Autodesk Inventor part; units mm, degrees
(part 3 of 4)
sketch "Sketch8" plane through (0, 0, 0.5) normal (0, 0, 1) x (1, 0, 0)
  circle A0 centre (6, 31.8) radius 0.9
  circle A1 centre (6, -31.8) radius 0.9
  line L0 (79.1, 6.35) -> (81.4, 6.35)
  line L1 (81.4, 6.35) -> (81.4, 7.9)
  line L2 (81.4, 7.9) -> (82.4, 7.9)
  line L3 (82.4, 7.9) -> (82.4, 5.35)
  line L4 (82.4, 5.35) -> (79.1, 5.35)
  line L5 (79.1, 5.35) -> (79.1, 6.35)
  line L6 (37.6, 36.65) -> (40.9, 36.65)
  line L7 (40.9, 36.65) -> (40.9, 35.65)
  line L8 (40.9, 35.65) -> (38.6, 35.65)
  line L9 (38.6, 35.65) -> (38.6, 34.1)
  line L10 (38.6, 34.1) -> (37.6, 34.1)
  line L11 (37.6, 34.1) -> (37.6, 36.65)
  line L12 (76.9, 36.65) -> (76.9, 35.65)
  line L13 (76.9, 35.65) -> (73.1, 35.65)
  line L14 (73.1, 35.65) -> (73.1, 36.65)
  line L15 (73.1, 36.65) -> (76.9, 36.65)
  line L16 (70.9, 6.35) -> (70.9, 5.35)
  line L17 (70.9, 5.35) -> (67.1, 5.35)
  line L18 (67.1, 5.35) -> (67.1, 6.35)
  line L19 (67.1, 6.35) -> (70.9, 6.35)
  line L20 (37.6, 16.1) -> (37.6, 19.9)
  line L21 (37.6, 19.9) -> (38.6, 19.9)
  line L22 (38.6, 19.9) -> (38.6, 16.1)
  line L23 (38.6, 16.1) -> (37.6, 16.1)
  line L24 (52.9, 36.65) -> (52.9, 35.65)
  line L25 (52.9, 35.65) -> (49.1, 35.65)
  line L26 (49.1, 35.65) -> (49.1, 36.65)
  line L27 (49.1, 36.65) -> (52.9, 36.65)
  line L28 (64.9, 36.65) -> (64.9, 35.65)
  line L29 (64.9, 35.65) -> (61.1, 35.65)
  line L30 (61.1, 35.65) -> (61.1, 36.65)
  line L31 (61.1, 36.65) -> (64.9, 36.65)
  line L32 (55.1, 6.35) -> (58.9, 6.35)
  line L33 (58.9, 6.35) -> (58.9, 5.35)
  line L34 (58.9, 5.35) -> (55.1, 5.35)
  line L35 (55.1, 5.35) -> (55.1, 6.35)
  line L36 (43.1, 6.35) -> (46.9, 6.35)
  line L37 (46.9, 6.35) -> (46.9, 5.35)
  line L38 (46.9, 5.35) -> (43.1, 5.35)
  line L39 (43.1, 5.35) -> (43.1, 6.35)
  line L40 (81.4, 25.9) -> (82.4, 25.9)
  line L41 (82.4, 25.9) -> (82.4, 22.1)
  line L42 (82.4, 22.1) -> (81.4, 22.1)
  line L43 (81.4, 22.1) -> (81.4, 25.9)
  line L44 (37.6, 28.1) -> (37.6, 31.9)
  line L45 (37.6, 31.9) -> (38.6, 31.9)
  line L46 (38.6, 31.9) -> (38.6, 28.1)
  line L47 (38.6, 28.1) -> (37.6, 28.1)
  line L48 (37.6, 10.1) -> (37.6, 13.9)
  line L49 (37.6, 13.9) -> (38.6, 13.9)
  line L50 (38.6, 13.9) -> (38.6, 10.1)
  line L51 (38.6, 10.1) -> (37.6, 10.1)
  line L52 (86.1, 14.6) -> (86.1, 13.25)
  line L53 (86.1, 13.25) -> (83.9, 13.25)
  line L54 (83.9, 13.25) -> (83.9, 14.6)
  line L55 (83.9, 14.6) -> (83.4, 14.6)
  line L56 (83.4, 14.6) -> (83.4, 15.4)
  line L57 (83.4, 15.4) -> (83.9, 15.4)
  line L58 (83.9, 15.4) -> (83.9, 16.75)
  line L59 (83.9, 16.75) -> (86.1, 16.75)
  line L60 (86.1, 16.75) -> (86.1, 15.4)
  line L61 (86.1, 15.4) -> (86.6, 15.4)
  line L62 (86.6, 15.4) -> (86.6, 14.6)
  line L63 (86.6, 14.6) -> (86.1, 14.6)
  line L64 (37.6, 22.1) -> (37.6, 25.9)
  line L65 (37.6, 25.9) -> (38.6, 25.9)
  line L66 (38.6, 25.9) -> (38.6, 22.1)
  line L67 (38.6, 22.1) -> (37.6, 22.1)
  line L68 (81.4, 31.9) -> (82.4, 31.9)
  line L69 (82.4, 31.9) -> (82.4, 28.1)
  line L70 (82.4, 28.1) -> (81.4, 28.1)
  line L71 (81.4, 28.1) -> (81.4, 31.9)
  line L72 (81.4, 13.9) -> (82.4, 13.9)
  line L73 (82.4, 13.9) -> (82.4, 10.1)
  line L74 (82.4, 10.1) -> (81.4, 10.1)
  line L75 (81.4, 10.1) -> (81.4, 13.9)
  line L76 (49.1, 6.35) -> (52.9, 6.35)
  line L77 (52.9, 6.35) -> (52.9, 5.35)
  line L78 (52.9, 5.35) -> (49.1, 5.35)
  line L79 (49.1, 5.35) -> (49.1, 6.35)
  line L80 (61.1, 6.35) -> (64.9, 6.35)
  line L81 (64.9, 6.35) -> (64.9, 5.35)
  line L82 (64.9, 5.35) -> (61.1, 5.35)
  line L83 (61.1, 5.35) -> (61.1, 6.35)
  line L84 (58.9, 36.65) -> (58.9, 35.65)
  line L85 (58.9, 35.65) -> (55.1, 35.65)
  line L86 (55.1, 35.65) -> (55.1, 36.65)
  line L87 (55.1, 36.65) -> (58.9, 36.65)
  line L88 (46.9, 36.65) -> (46.9, 35.65)
  line L89 (46.9, 35.65) -> (43.1, 35.65)
  line L90 (43.1, 35.65) -> (43.1, 36.65)
  line L91 (43.1, 36.65) -> (46.9, 36.65)
  line L92 (81.4, 19.9) -> (82.4, 19.9)
  line L93 (82.4, 19.9) -> (82.4, 16.1)
  line L94 (82.4, 16.1) -> (81.4, 16.1)
  line L95 (81.4, 16.1) -> (81.4, 19.9)
  line L96 (73.1, 6.35) -> (76.9, 6.35)
  line L97 (76.9, 6.35) -> (76.9, 5.35)
  line L98 (76.9, 5.35) -> (73.1, 5.35)
  line L99 (73.1, 5.35) -> (73.1, 6.35)
  line L100 (70.9, 36.65) -> (70.9, 35.65)
  line L101 (70.9, 35.65) -> (67.1, 35.65)
  line L102 (67.1, 35.65) -> (67.1, 36.65)
  line L103 (67.1, 36.65) -> (70.9, 36.65)
  line L104 (37.6, 5.35) -> (37.6, 7.9)
  line L105 (37.6, 7.9) -> (38.6, 7.9)
  line L106 (38.6, 7.9) -> (38.6, 6.35)
  line L107 (38.6, 6.35) -> (40.9, 6.35)
  line L108 (40.9, 6.35) -> (40.9, 5.35)
  line L109 (40.9, 5.35) -> (37.6, 5.35)
  line L110 (79.1, 35.65) -> (79.1, 36.65)
  line L111 (79.1, 36.65) -> (82.4, 36.65)
  line L112 (82.4, 36.65) -> (82.4, 34.1)
  line L113 (82.4, 34.1) -> (81.4, 34.1)
  line L114 (81.4, 34.1) -> (81.4, 35.65)
  line L115 (81.4, 35.65) -> (79.1, 35.65)
  line L116 (79.1, -33.65) -> (81.4, -33.65)
  line L117 (81.4, -33.65) -> (81.4, -32.1)
  line L118 (81.4, -32.1) -> (82.4, -32.1)
  line L119 (82.4, -32.1) -> (82.4, -34.65)
  line L120 (82.4, -34.65) -> (79.1, -34.65)
  line L121 (79.1, -34.65) -> (79.1, -33.65)
  line L122 (37.6, -3.35) -> (40.9, -3.35)
  line L123 (40.9, -3.35) -> (40.9, -4.35)
  line L124 (40.9, -4.35) -> (38.6, -4.35)
  line L125 (38.6, -4.35) -> (38.6, -5.9)
  line L126 (38.6, -5.9) -> (37.6, -5.9)
  line L127 (37.6, -5.9) -> (37.6, -3.35)
  line L128 (76.9, -3.35) -> (76.9, -4.35)
  line L129 (76.9, -4.35) -> (73.1, -4.35)
  line L130 (73.1, -4.35) -> (73.1, -3.35)
  line L131 (73.1, -3.35) -> (76.9, -3.35)
  line L132 (70.9, -33.65) -> (70.9, -34.65)
  line L133 (70.9, -34.65) -> (67.1, -34.65)
  line L134 (67.1, -34.65) -> (67.1, -33.65)
  line L135 (67.1, -33.65) -> (70.9, -33.65)
  line L136 (37.6, -23.9) -> (37.6, -20.1)
  line L137 (37.6, -20.1) -> (38.6, -20.1)
  line L138 (38.6, -20.1) -> (38.6, -23.9)
  line L139 (38.6, -23.9) -> (37.6, -23.9)
  line L140 (52.9, -3.35) -> (52.9, -4.35)
  line L141 (52.9, -4.35) -> (49.1, -4.35)
  line L142 (49.1, -4.35) -> (49.1, -3.35)
  line L143 (49.1, -3.35) -> (52.9, -3.35)
  line L144 (64.9, -3.35) -> (64.9, -4.35)
  line L145 (64.9, -4.35) -> (61.1, -4.35)
  line L146 (61.1, -4.35) -> (61.1, -3.35)
  line L147 (61.1, -3.35) -> (64.9, -3.35)
  line L148 (55.1, -33.65) -> (58.9, -33.65)
  line L149 (58.9, -33.65) -> (58.9, -34.65)
  line L150 (58.9, -34.65) -> (55.1, -34.65)
  line L151 (55.1, -34.65) -> (55.1, -33.65)
  line L152 (43.1, -33.65) -> (46.9, -33.65)
  line L153 (46.9, -33.65) -> (46.9, -34.65)
  line L154 (46.9, -34.65) -> (43.1, -34.65)
  line L155 (43.1, -34.65) -> (43.1, -33.65)
  line L156 (81.4, -14.1) -> (82.4, -14.1)
  line L157 (82.4, -14.1) -> (82.4, -17.9)
  line L158 (82.4, -17.9) -> (81.4, -17.9)
  line L159 (81.4, -17.9) -> (81.4, -14.1)
  line L160 (37.6, -11.9) -> (37.6, -8.1)
  line L161 (37.6, -8.1) -> (38.6, -8.1)
  line L162 (38.6, -8.1) -> (38.6, -11.9)
  line L163 (38.6, -11.9) -> (37.6, -11.9)
  line L164 (37.6, -29.9) -> (37.6, -26.1)
  line L165 (37.6, -26.1) -> (38.6, -26.1)
  line L166 (38.6, -26.1) -> (38.6, -29.9)
  line L167 (38.6, -29.9) -> (37.6, -29.9)
  line L168 (86.1, -25.4) -> (86.1, -26.75)
  line L169 (86.1, -26.75) -> (83.9, -26.75)
  line L170 (83.9, -26.75) -> (83.9, -25.4)
  line L171 (83.9, -25.4) -> (83.4, -25.4)
  line L172 (83.4, -25.4) -> (83.4, -24.6)
  line L173 (83.4, -24.6) -> (83.9, -24.6)
  line L174 (83.9, -24.6) -> (83.9, -23.25)
  line L175 (83.9, -23.25) -> (86.1, -23.25)
  line L176 (86.1, -23.25) -> (86.1, -24.6)
  line L177 (86.1, -24.6) -> (86.6, -24.6)
  line L178 (86.6, -24.6) -> (86.6, -25.4)
  line L179 (86.6, -25.4) -> (86.1, -25.4)
  line L180 (37.6, -17.9) -> (37.6, -14.1)
  line L181 (37.6, -14.1) -> (38.6, -14.1)
  line L182 (38.6, -14.1) -> (38.6, -17.9)
  line L183 (38.6, -17.9) -> (37.6, -17.9)
  line L184 (81.4, -8.1) -> (82.4, -8.1)
  line L185 (82.4, -8.1) -> (82.4, -11.9)
  line L186 (82.4, -11.9) -> (81.4, -11.9)
  line L187 (81.4, -11.9) -> (81.4, -8.1)
  line L188 (81.4, -26.1) -> (82.4, -26.1)
  line L189 (82.4, -26.1) -> (82.4, -29.9)
  line L190 (82.4, -29.9) -> (81.4, -29.9)
  line L191 (81.4, -29.9) -> (81.4, -26.1)
  line L192 (49.1, -33.65) -> (52.9, -33.65)
  line L193 (52.9, -33.65) -> (52.9, -34.65)
  line L194 (52.9, -34.65) -> (49.1, -34.65)
  line L195 (49.1, -34.65) -> (49.1, -33.65)
  line L196 (61.1, -33.65) -> (64.9, -33.65)
  line L197 (64.9, -33.65) -> (64.9, -34.65)
  line L198 (64.9, -34.65) -> (61.1, -34.65)
  line L199 (61.1, -34.65) -> (61.1, -33.65)
  line L200 (58.9, -3.35) -> (58.9, -4.35)
  line L201 (58.9, -4.35) -> (55.1, -4.35)
  line L202 (55.1, -4.35) -> (55.1, -3.35)
  line L203 (55.1, -3.35) -> (58.9, -3.35)
  line L204 (46.9, -3.35) -> (46.9, -4.35)
  line L205 (46.9, -4.35) -> (43.1, -4.35)
  line L206 (43.1, -4.35) -> (43.1, -3.35)
  line L207 (43.1, -3.35) -> (46.9, -3.35)
  line L208 (81.4, -20.1) -> (82.4, -20.1)
  line L209 (82.4, -20.1) -> (82.4, -23.9)
  line L210 (82.4, -23.9) -> (81.4, -23.9)
  line L211 (81.4, -23.9) -> (81.4, -20.1)
  line L212 (73.1, -33.65) -> (76.9, -33.65)
  line L213 (76.9, -33.65) -> (76.9, -34.65)
  line L214 (76.9, -34.65) -> (73.1, -34.65)
  line L215 (73.1, -34.65) -> (73.1, -33.65)
  line L216 (70.9, -3.35) -> (70.9, -4.35)
  line L217 (70.9, -4.35) -> (67.1, -4.35)
  line L218 (67.1, -4.35) -> (67.1, -3.35)
  line L219 (67.1, -3.35) -> (70.9, -3.35)
  line L220 (37.6, -34.65) -> (37.6, -32.1)
  line L221 (37.6, -32.1) -> (38.6, -32.1)
  line L222 (38.6, -32.1) -> (38.6, -33.65)
  line L223 (38.6, -33.65) -> (40.9, -33.65)
  line L224 (40.9, -33.65) -> (40.9, -34.65)
  line L225 (40.9, -34.65) -> (37.6, -34.65)
  line L226 (79.1, -4.35) -> (79.1, -3.35)
  line L227 (79.1, -3.35) -> (82.4, -3.35)
  line L228 (82.4, -3.35) -> (82.4, -5.9)
  line L229 (82.4, -5.9) -> (81.4, -5.9)
  line L230 (81.4, -5.9) -> (81.4, -4.35)
  line L231 (81.4, -4.35) -> (79.1, -4.35)
  line L232 (31.7, -27.5) -> (30.7, -27.5)
  line L233 (30.7, -27.5) -> (30.7, -25)
  line L234 (30.7, -25) -> (31.7, -25)
  line L235 (31.7, -25) -> (31.7, -27.5)
  line L236 (26.62, -27.5) -> (25.62, -27.5)
  line L237 (25.62, -27.5) -> (25.62, -25)
  line L238 (25.62, -25) -> (26.62, -25)
  line L239 (26.62, -25) -> (26.62, -27.5)
  line L240 (21.54, -27.5) -> (20.54, -27.5)
  line L241 (20.54, -27.5) -> (20.54, -25)
  line L242 (20.54, -25) -> (21.54, -25)
  line L243 (21.54, -25) -> (21.54, -27.5)
  line L244 (14.5, 8.6) -> (14.5, 9.75)
  line L245 (14.5, 9.75) -> (15.9, 9.75)
  line L246 (15.9, 9.75) -> (15.9, 8.6)
  line L247 (15.9, 8.6) -> (14.5, 8.6)
  line L248 (17.5, 7) -> (17.5, 8.15)
  line L249 (17.5, 8.15) -> (18.9, 8.15)
  line L250 (18.9, 8.15) -> (18.9, 7)
  line L251 (18.9, 7) -> (17.5, 7)
  line L252 (23.4831, 10.3536) -> (22.3831, 10.3536)
  line L253 (22.3831, 10.3536) -> (22.3831, 11.4536)
  line L254 (22.3831, 11.4536) -> (23.4831, 11.4536)
  line L255 (23.4831, 11.4536) -> (23.4831, 10.3536)
  line L256 (18.75, 11.78) -> (17.65, 11.78)
  line L257 (17.65, 11.78) -> (17.65, 12.88)
  line L258 (17.65, 12.88) -> (18.75, 12.88)
  line L259 (18.75, 12.88) -> (18.75, 11.78)
  line L260 (15.75, 11.78) -> (14.65, 11.78)
  line L261 (14.65, 11.78) -> (14.65, 12.88)
  line L262 (14.65, 12.88) -> (15.75, 12.88)
  line L263 (15.75, 12.88) -> (15.75, 11.78)
  line L264 (23.9, 6.8) -> (23.9, 7.9)
  line L265 (23.9, 7.9) -> (25, 7.9)
  line L266 (25, 7.9) -> (25, 6.8)
  line L267 (25, 6.8) -> (23.9, 6.8)
  line L268 (26.8, -3.9) -> (27.9, -3.9)
  line L269 (27.9, -3.9) -> (27.9, -5)
  line L270 (27.9, -5) -> (26.8, -5)
  line L271 (26.8, -5) -> (26.8, -3.9)
  line L272 (16.1, -6.8) -> (16.1, -7.9)
  line L273 (16.1, -7.9) -> (15, -7.9)
  line L274 (15, -7.9) -> (15, -6.8)
  line L275 (15, -6.8) -> (16.1, -6.8)
  line L276 (13.2, 5) -> (13.2, 3.9)
  line L277 (13.2, 3.9) -> (12.1, 3.9)
  line L278 (12.1, 3.9) -> (12.1, 5)
  line L279 (12.1, 5) -> (13.2, 5)
  line L280 (26.35, -3.6) -> (26.35, -3.9)
  line L281 (26.35, -3.9) -> (25.15, -3.9)
  line L282 (25.15, -3.9) -> (25.15, -3.6)
  line L283 (25.15, -3.6) -> (26.35, -3.6)
  line L284 (26.35, -3.1) -> (26.35, -3.4)
  line L285 (26.35, -3.4) -> (25.15, -3.4)
  line L286 (25.15, -3.4) -> (25.15, -3.1)
  line L287 (25.15, -3.1) -> (26.35, -3.1)
  line L288 (26.35, -2.6) -> (26.35, -2.9)
  line L289 (26.35, -2.9) -> (25.15, -2.9)
  line L290 (25.15, -2.9) -> (25.15, -2.6)
  line L291 (25.15, -2.6) -> (26.35, -2.6)
  line L292 (26.35, -2.1) -> (26.35, -2.4)
  line L293 (26.35, -2.4) -> (25.15, -2.4)
  line L294 (25.15, -2.4) -> (25.15, -2.1)
  line L295 (25.15, -2.1) -> (26.35, -2.1)
  line L296 (26.35, -1.6) -> (26.35, -1.9)
  line L297 (26.35, -1.9) -> (25.15, -1.9)
  line L298 (25.15, -1.9) -> (25.15, -1.6)
  line L299 (25.15, -1.6) -> (26.35, -1.6)
  line L300 (26.35, -1.1) -> (26.35, -1.4)
  line L301 (26.35, -1.4) -> (25.15, -1.4)
  line L302 (25.15, -1.4) -> (25.15, -1.1)
  line L303 (25.15, -1.1) -> (26.35, -1.1)
  line L304 (26.35, -0.6) -> (26.35, -0.9)
  line L305 (26.35, -0.9) -> (25.15, -0.9)
  line L306 (25.15, -0.9) -> (25.15, -0.6)
  line L307 (25.15, -0.6) -> (26.35, -0.6)
  line L308 (26.35, -0.1) -> (26.35, -0.4)
  line L309 (26.35, -0.4) -> (25.15, -0.4)
  line L310 (25.15, -0.4) -> (25.15, -0.1)
  line L311 (25.15, -0.1) -> (26.35, -0.1)
  line L312 (26.35, 0.4) -> (26.35, 0.1)
  line L313 (26.35, 0.1) -> (25.15, 0.1)
  line L314 (25.15, 0.1) -> (25.15, 0.4)
  line L315 (25.15, 0.4) -> (26.35, 0.4)
  line L316 (26.35, 0.9) -> (26.35, 0.6)
  line L317 (26.35, 0.6) -> (25.15, 0.6)
  line L318 (25.15, 0.6) -> (25.15, 0.9)
  line L319 (25.15, 0.9) -> (26.35, 0.9)
  line L320 (26.35, 1.4) -> (26.35, 1.1)
  line L321 (26.35, 1.1) -> (25.15, 1.1)
  line L322 (25.15, 1.1) -> (25.15, 1.4)
  line L323 (25.15, 1.4) -> (26.35, 1.4)
  line L324 (26.35, 1.9) -> (26.35, 1.6)
  line L325 (26.35, 1.6) -> (25.15, 1.6)
  line L326 (25.15, 1.6) -> (25.15, 1.9)
  line L327 (25.15, 1.9) -> (26.35, 1.9)
  line L328 (26.35, 2.4) -> (26.35, 2.1)
  line L329 (26.35, 2.1) -> (25.15, 2.1)
  line L330 (25.15, 2.1) -> (25.15, 2.4)
  line L331 (25.15, 2.4) -> (26.35, 2.4)
  line L332 (26.35, 2.9) -> (26.35, 2.6)
  line L333 (26.35, 2.6) -> (25.15, 2.6)
  line L334 (25.15, 2.6) -> (25.15, 2.9)
  line L335 (25.15, 2.9) -> (26.35, 2.9)
  line L336 (26.35, 3.4) -> (26.35, 3.1)
  line L337 (26.35, 3.1) -> (25.15, 3.1)
  line L338 (25.15, 3.1) -> (25.15, 3.4)
  line L339 (25.15, 3.4) -> (26.35, 3.4)
  line L340 (14.85, 3.9) -> (14.85, 3.6)
  line L341 (14.85, 3.6) -> (13.65, 3.6)
  line L342 (13.65, 3.6) -> (13.65, 3.9)
  line L343 (13.65, 3.9) -> (14.85, 3.9)
  line L344 (23.9, -5.15) -> (23.9, -6.35)
  line L345 (23.9, -6.35) -> (23.6, -6.35)
  line L346 (23.6, -6.35) -> (23.6, -5.15)
  line L347 (23.6, -5.15) -> (23.9, -5.15)
  line L348 (23.4, -5.15) -> (23.4, -6.35)
  line L349 (23.4, -6.35) -> (23.1, -6.35)
  line L350 (23.1, -6.35) -> (23.1, -5.15)
  line L351 (23.1, -5.15) -> (23.4, -5.15)
  line L352 (22.9, -5.15) -> (22.9, -6.35)
  line L353 (22.9, -6.35) -> (22.6, -6.35)
  line L354 (22.6, -6.35) -> (22.6, -5.15)
  line L355 (22.6, -5.15) -> (22.9, -5.15)
  line L356 (22.4, -5.15) -> (22.4, -6.35)
  line L357 (22.4, -6.35) -> (22.1, -6.35)
  line L358 (22.1, -6.35) -> (22.1, -5.15)
  line L359 (22.1, -5.15) -> (22.4, -5.15)
  line L360 (21.9, -5.15) -> (21.9, -6.35)
  line L361 (21.9, -6.35) -> (21.6, -6.35)
  line L362 (21.6, -6.35) -> (21.6, -5.15)
  line L363 (21.6, -5.15) -> (21.9, -5.15)
  line L364 (21.4, -5.15) -> (21.4, -6.35)
  line L365 (21.4, -6.35) -> (21.1, -6.35)
  line L366 (21.1, -6.35) -> (21.1, -5.15)
  line L367 (21.1, -5.15) -> (21.4, -5.15)
  line L368 (20.9, -5.15) -> (20.9, -6.35)
  line L369 (20.9, -6.35) -> (20.6, -6.35)
  line L370 (20.6, -6.35) -> (20.6, -5.15)
  line L371 (20.6, -5.15) -> (20.9, -5.15)
  line L372 (20.4, -5.15) -> (20.4, -6.35)
  line L373 (20.4, -6.35) -> (20.1, -6.35)
  line L374 (20.1, -6.35) -> (20.1, -5.15)
  line L375 (20.1, -5.15) -> (20.4, -5.15)
  line L376 (19.9, -5.15) -> (19.9, -6.35)
  line L377 (19.9, -6.35) -> (19.6, -6.35)
  line L378 (19.6, -6.35) -> (19.6, -5.15)
  line L379 (19.6, -5.15) -> (19.9, -5.15)
  line L380 (19.4, -5.15) -> (19.4, -6.35)
  line L381 (19.4, -6.35) -> (19.1, -6.35)
  line L382 (19.1, -6.35) -> (19.1, -5.15)
  line L383 (19.1, -5.15) -> (19.4, -5.15)
  line L384 (18.9, -5.15) -> (18.9, -6.35)
  line L385 (18.9, -6.35) -> (18.6, -6.35)
  line L386 (18.6, -6.35) -> (18.6, -5.15)
  line L387 (18.6, -5.15) -> (18.9, -5.15)
  line L388 (18.4, -5.15) -> (18.4, -6.35)
  line L389 (18.4, -6.35) -> (18.1, -6.35)
  line L390 (18.1, -6.35) -> (18.1, -5.15)
  line L391 (18.1, -5.15) -> (18.4, -5.15)
  line L392 (17.9, -5.15) -> (17.9, -6.35)
  line L393 (17.9, -6.35) -> (17.6, -6.35)
  line L394 (17.6, -6.35) -> (17.6, -5.15)
  line L395 (17.6, -5.15) -> (17.9, -5.15)
  line L396 (17.4, -5.15) -> (17.4, -6.35)
  line L397 (17.4, -6.35) -> (17.1, -6.35)
  line L398 (17.1, -6.35) -> (17.1, -5.15)
  line L399 (17.1, -5.15) -> (17.4, -5.15)
  line L400 (16.9, -5.15) -> (16.9, -6.35)
  line L401 (16.9, -6.35) -> (16.6, -6.35)
  line L402 (16.6, -6.35) -> (16.6, -5.15)
  line L403 (16.6, -5.15) -> (16.9, -5.15)
  line L404 (16.4, -5.15) -> (16.4, -6.35)
  line L405 (16.4, -6.35) -> (16.1, -6.35)
  line L406 (16.1, -6.35) -> (16.1, -5.15)
  line L407 (16.1, -5.15) -> (16.4, -5.15)
  line L408 (16.4, 6.35) -> (16.4, 5.15)
  line L409 (16.4, 5.15) -> (16.1, 5.15)
  line L410 (16.1, 5.15) -> (16.1, 6.35)
  line L411 (16.1, 6.35) -> (16.4, 6.35)
  line L412 (16.9, 6.35) -> (16.9, 5.15)
  line L413 (16.9, 5.15) -> (16.6, 5.15)
  line L414 (16.6, 5.15) -> (16.6, 6.35)
  line L415 (16.6, 6.35) -> (16.9, 6.35)
  line L416 (17.4, 6.35) -> (17.4, 5.15)
  line L417 (17.4, 5.15) -> (17.1, 5.15)
  line L418 (17.1, 5.15) -> (17.1, 6.35)
  line L419 (17.1, 6.35) -> (17.4, 6.35)
  line L420 (17.9, 6.35) -> (17.9, 5.15)
  line L421 (17.9, 5.15) -> (17.6, 5.15)
  line L422 (17.6, 5.15) -> (17.6, 6.35)
  line L423 (17.6, 6.35) -> (17.9, 6.35)
  line L424 (18.4, 6.35) -> (18.4, 5.15)
  line L425 (18.4, 5.15) -> (18.1, 5.15)
  line L426 (18.1, 5.15) -> (18.1, 6.35)
  line L427 (18.1, 6.35) -> (18.4, 6.35)
  line L428 (18.9, 6.35) -> (18.9, 5.15)
  line L429 (18.9, 5.15) -> (18.6, 5.15)
  line L430 (18.6, 5.15) -> (18.6, 6.35)
  line L431 (18.6, 6.35) -> (18.9, 6.35)
  line L432 (19.4, 6.35) -> (19.4, 5.15)
  line L433 (19.4, 5.15) -> (19.1, 5.15)
  line L434 (19.1, 5.15) -> (19.1, 6.35)
  line L435 (19.1, 6.35) -> (19.4, 6.35)
  line L436 (19.9, 6.35) -> (19.9, 5.15)
  line L437 (19.9, 5.15) -> (19.6, 5.15)
  line L438 (19.6, 5.15) -> (19.6, 6.35)
  line L439 (19.6, 6.35) -> (19.9, 6.35)
  line L440 (20.4, 6.35) -> (20.4, 5.15)
  line L441 (20.4, 5.15) -> (20.1, 5.15)
  line L442 (20.1, 5.15) -> (20.1, 6.35)
  line L443 (20.1, 6.35) -> (20.4, 6.35)
  line L444 (20.9, 6.35) -> (20.9, 5.15)
  line L445 (20.9, 5.15) -> (20.6, 5.15)
  line L446 (20.6, 5.15) -> (20.6, 6.35)
  line L447 (20.6, 6.35) -> (20.9, 6.35)
  line L448 (21.4, 6.35) -> (21.4, 5.15)
  line L449 (21.4, 5.15) -> (21.1, 5.15)
  line L450 (21.1, 5.15) -> (21.1, 6.35)
  line L451 (21.1, 6.35) -> (21.4, 6.35)
  line L452 (21.9, 6.35) -> (21.9, 5.15)
  line L453 (21.9, 5.15) -> (21.6, 5.15)
  line L454 (21.6, 5.15) -> (21.6, 6.35)
  line L455 (21.6, 6.35) -> (21.9, 6.35)
  line L456 (22.4, 6.35) -> (22.4, 5.15)
  line L457 (22.4, 5.15) -> (22.1, 5.15)
  line L458 (22.1, 5.15) -> (22.1, 6.35)
  line L459 (22.1, 6.35) -> (22.4, 6.35)
  line L460 (22.9, 6.35) -> (22.9, 5.15)
  line L461 (22.9, 5.15) -> (22.6, 5.15)
  line L462 (22.6, 5.15) -> (22.6, 6.35)
  line L463 (22.6, 6.35) -> (22.9, 6.35)
  line L464 (23.4, 6.35) -> (23.4, 5.15)
  line L465 (23.4, 5.15) -> (23.1, 5.15)
  line L466 (23.1, 5.15) -> (23.1, 6.35)
  line L467 (23.1, 6.35) -> (23.4, 6.35)
  line L468 (23.9, 6.35) -> (23.9, 5.15)
  line L469 (23.9, 5.15) -> (23.6, 5.15)
  line L470 (23.6, 5.15) -> (23.6, 6.35)
  line L471 (23.6, 6.35) -> (23.9, 6.35)
  line L472 (26.35, 3.9) -> (26.35, 3.6)
  line L473 (26.35, 3.6) -> (25.15, 3.6)
  line L474 (25.15, 3.6) -> (25.15, 3.9)
  line L475 (25.15, 3.9) -> (26.35, 3.9)
  line L476 (14.85, 3.1) -> (13.65, 3.1)
  line L477 (13.65, 3.1) -> (13.65, 3.4)
  line L478 (13.65, 3.4) -> (14.85, 3.4)
  line L479 (14.85, 3.4) -> (14.85, 3.1)
  line L480 (14.85, 2.6) -> (13.65, 2.6)
  line L481 (13.65, 2.6) -> (13.65, 2.9)
  line L482 (13.65, 2.9) -> (14.85, 2.9)
  line L483 (14.85, 2.9) -> (14.85, 2.6)
  line L484 (14.85, 2.1) -> (13.65, 2.1)
  line L485 (13.65, 2.1) -> (13.65, 2.4)
  line L486 (13.65, 2.4) -> (14.85, 2.4)
  line L487 (14.85, 2.4) -> (14.85, 2.1)
  line L488 (14.85, 1.6) -> (13.65, 1.6)
  line L489 (13.65, 1.6) -> (13.65, 1.9)
  line L490 (13.65, 1.9) -> (14.85, 1.9)
  line L491 (14.85, 1.9) -> (14.85, 1.6)
  line L492 (14.85, 1.1) -> (13.65, 1.1)
  line L493 (13.65, 1.1) -> (13.65, 1.4)
  line L494 (13.65, 1.4) -> (14.85, 1.4)
  line L495 (14.85, 1.4) -> (14.85, 1.1)
  line L496 (14.85, 0.6) -> (13.65, 0.6)
  line L497 (13.65, 0.6) -> (13.65, 0.9)
  line L498 (13.65, 0.9) -> (14.85, 0.9)
  line L499 (14.85, 0.9) -> (14.85, 0.6)
  line L500 (14.85, 0.1) -> (13.65, 0.1)
  line L501 (13.65, 0.1) -> (13.65, 0.4)
  line L502 (13.65, 0.4) -> (14.85, 0.4)
  line L503 (14.85, 0.4) -> (14.85, 0.1)
  line L504 (14.85, -0.4) -> (13.65, -0.4)
  line L505 (13.65, -0.4) -> (13.65, -0.1)
  line L506 (13.65, -0.1) -> (14.85, -0.1)
  line L507 (14.85, -0.1) -> (14.85, -0.4)
  line L508 (14.85, -0.9) -> (13.65, -0.9)
  line L509 (13.65, -0.9) -> (13.65, -0.6)
  line L510 (13.65, -0.6) -> (14.85, -0.6)
  line L511 (14.85, -0.6) -> (14.85, -0.9)
  line L512 (14.85, -1.4) -> (13.65, -1.4)
  line L513 (13.65, -1.4) -> (13.65, -1.1)
  line L514 (13.65, -1.1) -> (14.85, -1.1)
  line L515 (14.85, -1.1) -> (14.85, -1.4)
  line L516 (14.85, -1.9) -> (13.65, -1.9)
  line L517 (13.65, -1.9) -> (13.65, -1.6)
  line L518 (13.65, -1.6) -> (14.85, -1.6)
  line L519 (14.85, -1.6) -> (14.85, -1.9)
  line L520 (14.85, -2.4) -> (13.65, -2.4)
  line L521 (13.65, -2.4) -> (13.65, -2.1)
  line L522 (13.65, -2.1) -> (14.85, -2.1)
  line L523 (14.85, -2.1) -> (14.85, -2.4)
  line L524 (14.85, -2.9) -> (13.65, -2.9)
  line L525 (13.65, -2.9) -> (13.65, -2.6)
  line L526 (13.65, -2.6) -> (14.85, -2.6)
  line L527 (14.85, -2.6) -> (14.85, -2.9)
  line L528 (14.85, -3.4) -> (13.65, -3.4)
  line L529 (13.65, -3.4) -> (13.65, -3.1)
  line L530 (13.65, -3.1) -> (14.85, -3.1)
  line L531 (14.85, -3.1) -> (14.85, -3.4)
  line L532 (14.85, -3.9) -> (13.65, -3.9)
  line L533 (13.65, -3.9) -> (13.65, -3.6)
  line L534 (13.65, -3.6) -> (14.85, -3.6)
  line L535 (14.85, -3.6) -> (14.85, -3.9)
  line L536 (13.2, 6.73) -> (13.2, 5.63)
  line L537 (13.2, 5.63) -> (12.1, 5.63)
  line L538 (12.1, 5.63) -> (12.1, 6.73)
  line L539 (12.1, 6.73) -> (13.2, 6.73)
  line L540 (14.37, -6.8) -> (14.37, -7.9)
  line L541 (14.37, -7.9) -> (13.27, -7.9)
  line L542 (13.27, -7.9) -> (13.27, -6.8)
  line L543 (13.27, -6.8) -> (14.37, -6.8)
  line L544 (26.8, -5.63) -> (27.9, -5.63)
  line L545 (27.9, -5.63) -> (27.9, -6.73)
  line L546 (27.9, -6.73) -> (26.8, -6.73)
  line L547 (26.8, -6.73) -> (26.8, -5.63)
  line L548 (25.63, 6.8) -> (25.63, 7.9)
  line L549 (25.63, 7.9) -> (26.73, 7.9)
  line L550 (26.73, 7.9) -> (26.73, 6.8)
  line L551 (26.73, 6.8) -> (25.63, 6.8)
  line L552 (15.75, 10.05) -> (14.65, 10.05)
  line L553 (14.65, 10.05) -> (14.65, 11.15)
  line L554 (14.65, 11.15) -> (15.75, 11.15)
  line L555 (15.75, 11.15) -> (15.75, 10.05)
  line L556 (18.75, 10.05) -> (17.65, 10.05)
  line L557 (17.65, 10.05) -> (17.65, 11.15)
  line L558 (17.65, 11.15) -> (18.75, 11.15)
  line L559 (18.75, 11.15) -> (18.75, 10.05)
  line L560 (25.2131, 10.3536) -> (24.1131, 10.3536)
  line L561 (24.1131, 10.3536) -> (24.1131, 11.4536)
  line L562 (24.1131, 11.4536) -> (25.2131, 11.4536)
  line L563 (25.2131, 11.4536) -> (25.2131, 10.3536)
  line L564 (18.9, 9.75) -> (18.9, 8.6)
  line L565 (18.9, 8.6) -> (17.5, 8.6)
  line L566 (17.5, 8.6) -> (17.5, 9.75)
  line L567 (17.5, 9.75) -> (18.9, 9.75)
  line L568 (14.5, 7) -> (14.5, 8.15)
  line L569 (14.5, 8.15) -> (15.9, 8.15)
  line L570 (15.9, 8.15) -> (15.9, 7)
  line L571 (15.9, 7) -> (14.5, 7)
  line L572 (19, -25) -> (19, -27.5)
  line L573 (19, -27.5) -> (18, -27.5)
  line L574 (18, -27.5) -> (18, -25)
  line L575 (18, -25) -> (19, -25)
  line L576 (24.08, -27.5) -> (23.08, -27.5)
  line L577 (23.08, -27.5) -> (23.08, -25)
  line L578 (23.08, -25) -> (24.08, -25)
  line L579 (24.08, -25) -> (24.08, -27.5)
  line L580 (29.16, -27.5) -> (28.16, -27.5)
  line L581 (28.16, -27.5) -> (28.16, -25)
  line L582 (28.16, -25) -> (29.16, -25)
  line L583 (29.16, -25) -> (29.16, -27.5)
  line L584 (2.8, -31.125) -> (2.8, -31.575)
  line L585 (2.8, -31.575) -> (0.25, -31.575)
  line L586 (0.25, -31.575) -> (0.25, -31.125)
  line L587 (0.25, -31.125) -> (2.8, -31.125)
  line L588 (2.8, -29.925) -> (2.8, -30.375)
  line L589 (2.8, -30.375) -> (0.25, -30.375)
  line L590 (0.25, -30.375) -> (0.25, -29.925)
  line L591 (0.25, -29.925) -> (2.8, -29.925)
  line L592 (2.8, -28.725) -> (2.8, -29.175)
  line L593 (2.8, -29.175) -> (0.25, -29.175)
  line L594 (0.25, -29.175) -> (0.25, -28.725)
  line L595 (0.25, -28.725) -> (2.8, -28.725)
  line L596 (2.8, -27.525) -> (2.8, -27.975)
  line L597 (2.8, -27.975) -> (0.25, -27.975)
  line L598 (0.25, -27.975) -> (0.25, -27.525)
  line L599 (0.25, -27.525) -> (2.8, -27.525)
  line L600 (2.8, -26.325) -> (2.8, -26.775)
  line L601 (2.8, -26.775) -> (0.25, -26.775)
  line L602 (0.25, -26.775) -> (0.25, -26.325)
  line L603 (0.25, -26.325) -> (2.8, -26.325)
  line L604 (2.8, -25.125) -> (2.8, -25.575)
  line L605 (2.8, -25.575) -> (0.25, -25.575)
  line L606 (0.25, -25.575) -> (0.25, -25.125)
  line L607 (0.25, -25.125) -> (2.8, -25.125)
  line L608 (2.8, -23.925) -> (2.8, -24.375)
  line L609 (2.8, -24.375) -> (0.25, -24.375)
  line L610 (0.25, -24.375) -> (0.25, -23.925)
  line L611 (0.25, -23.925) -> (2.8, -23.925)
  line L612 (2.8, -22.725) -> (2.8, -23.175)
  line L613 (2.8, -23.175) -> (0.25, -23.175)
  line L614 (0.25, -23.175) -> (0.25, -22.725)
  line L615 (0.25, -22.725) -> (2.8, -22.725)
  line L616 (2.8, -21.525) -> (2.8, -21.975)
  line L617 (2.8, -21.975) -> (0.25, -21.975)
  line L618 (0.25, -21.975) -> (0.25, -21.525)
  line L619 (0.25, -21.525) -> (2.8, -21.525)
  line L620 (2.8, -20.325) -> (2.8, -20.775)
  line L621 (2.8, -20.775) -> (0.25, -20.775)
  line L622 (0.25, -20.775) -> (0.25, -20.325)
  line L623 (0.25, -20.325) -> (2.8, -20.325)
  line L624 (2.8, -19.125) -> (2.8, -19.575)
  line L625 (2.8, -19.575) -> (0.25, -19.575)
  line L626 (0.25, -19.575) -> (0.25, -19.125)
  line L627 (0.25, -19.125) -> (2.8, -19.125)
  line L628 (2.8, -17.925) -> (2.8, -18.375)
  line L629 (2.8, -18.375) -> (0.25, -18.375)
  line L630 (0.25, -18.375) -> (0.25, -17.925)
  line L631 (0.25, -17.925) -> (2.8, -17.925)
  line L632 (2.8, -16.725) -> (2.8, -17.175)
  line L633 (2.8, -17.175) -> (0.25, -17.175)
  line L634 (0.25, -17.175) -> (0.25, -16.725)
  line L635 (0.25, -16.725) -> (2.8, -16.725)
  line L636 (2.8, -15.525) -> (2.8, -15.975)
  line L637 (2.8, -15.975) -> (0.25, -15.975)
  line L638 (0.25, -15.975) -> (0.25, -15.525)
  line L639 (0.25, -15.525) -> (2.8, -15.525)
  line L640 (2.8, -14.325) -> (2.8, -14.775)
  line L641 (2.8, -14.775) -> (0.25, -14.775)
  line L642 (0.25, -14.775) -> (0.25, -14.325)
  line L643 (0.25, -14.325) -> (2.8, -14.325)
  line L644 (2.8, -13.125) -> (2.8, -13.575)
  line L645 (2.8, -13.575) -> (0.25, -13.575)
  line L646 (0.25, -13.575) -> (0.25, -13.125)
  line L647 (0.25, -13.125) -> (2.8, -13.125)
  line L648 (2.8, -11.925) -> (2.8, -12.375)
  line L649 (2.8, -12.375) -> (0.25, -12.375)
  line L650 (0.25, -12.375) -> (0.25, -11.925)
  line L651 (0.25, -11.925) -> (2.8, -11.925)
  line L652 (2.8, -10.725) -> (2.8, -11.175)
  line L653 (2.8, -11.175) -> (0.25, -11.175)
  line L654 (0.25, -11.175) -> (0.25, -10.725)
  line L655 (0.25, -10.725) -> (2.8, -10.725)
  line L656 (2.8, -9.525) -> (2.8, -9.975)
  line L657 (2.8, -9.975) -> (0.25, -9.975)
  line L658 (0.25, -9.975) -> (0.25, -9.525)
  line L659 (0.25, -9.525) -> (2.8, -9.525)
  line L660 (2.8, -8.325) -> (2.8, -8.775)
  line L661 (2.8, -8.775) -> (0.25, -8.775)
  line L662 (0.25, -8.775) -> (0.25, -8.325)
  line L663 (0.25, -8.325) -> (2.8, -8.325)
  line L664 (2.8, -7.125) -> (2.8, -7.575)
  line L665 (2.8, -7.575) -> (0.25, -7.575)
  line L666 (0.25, -7.575) -> (0.25, -7.125)
  line L667 (0.25, -7.125) -> (2.8, -7.125)
  line L668 (2.8, -5.925) -> (2.8, -6.375)
  line L669 (2.8, -6.375) -> (0.25, -6.375)
  line L670 (0.25, -6.375) -> (0.25, -5.925)
  line L671 (0.25, -5.925) -> (2.8, -5.925)
  line L672 (2.8, -4.725) -> (2.8, -5.175)
  line L673 (2.8, -5.175) -> (0.25, -5.175)
  line L674 (0.25, -5.175) -> (0.25, -4.725)
  line L675 (0.25, -4.725) -> (2.8, -4.725)
  line L676 (2.8, -3.525) -> (2.8, -3.975)
  line L677 (2.8, -3.975) -> (0.25, -3.975)
  line L678 (0.25, -3.975) -> (0.25, -3.525)
  line L679 (0.25, -3.525) -> (2.8, -3.525)
  line L680 (2.8, -2.325) -> (2.8, -2.775)
  line L681 (2.8, -2.775) -> (0.25, -2.775)
  line L682 (0.25, -2.775) -> (0.25, -2.325)
  line L683 (0.25, -2.325) -> (2.8, -2.325)
  line L684 (2.8, -1.125) -> (2.8, -1.575)
  line L685 (2.8, -1.575) -> (0.25, -1.575)
  line L686 (0.25, -1.575) -> (0.25, -1.125)
  line L687 (0.25, -1.125) -> (2.8, -1.125)
  line L688 (2.8, 0.075) -> (2.8, -0.375)
  line L689 (2.8, -0.375) -> (0.25, -0.375)
  line L690 (0.25, -0.375) -> (0.25, 0.075)
  line L691 (0.25, 0.075) -> (2.8, 0.075)
  line L692 (2.8, 1.275) -> (2.8, 0.825)
  line L693 (2.8, 0.825) -> (0.25, 0.825)
  line L694 (0.25, 0.825) -> (0.25, 1.275)
  line L695 (0.25, 1.275) -> (2.8, 1.275)
  line L696 (2.8, 2.475) -> (2.8, 2.025)
  line L697 (2.8, 2.025) -> (0.25, 2.025)
  line L698 (0.25, 2.025) -> (0.25, 2.475)
  line L699 (0.25, 2.475) -> (2.8, 2.475)
  line L700 (2.8, 3.675) -> (2.8, 3.225)
  line L701 (2.8, 3.225) -> (0.25, 3.225)
  line L702 (0.25, 3.225) -> (0.25, 3.675)
  line L703 (0.25, 3.675) -> (2.8, 3.675)
  line L704 (2.8, 4.875) -> (2.8, 4.425)
  line L705 (2.8, 4.425) -> (0.25, 4.425)
  line L706 (0.25, 4.425) -> (0.25, 4.875)
  line L707 (0.25, 4.875) -> (2.8, 4.875)
  line L708 (2.8, 6.075) -> (2.8, 5.625)
  line L709 (2.8, 5.625) -> (0.25, 5.625)
  line L710 (0.25, 5.625) -> (0.25, 6.075)
  line L711 (0.25, 6.075) -> (2.8, 6.075)
  line L712 (2.8, 7.275) -> (2.8, 6.825)
  line L713 (2.8, 6.825) -> (0.25, 6.825)
  line L714 (0.25, 6.825) -> (0.25, 7.275)
  line L715 (0.25, 7.275) -> (2.8, 7.275)
  line L716 (2.8, 8.475) -> (2.8, 8.025)
  line L717 (2.8, 8.025) -> (0.25, 8.025)
  line L718 (0.25, 8.025) -> (0.25, 8.475)
  line L719 (0.25, 8.475) -> (2.8, 8.475)
  line L720 (2.8, 9.675) -> (2.8, 9.225)
  line L721 (2.8, 9.225) -> (0.25, 9.225)
  line L722 (0.25, 9.225) -> (0.25, 9.675)
  line L723 (0.25, 9.675) -> (2.8, 9.675)
  line L724 (2.8, 10.875) -> (2.8, 10.425)
  line L725 (2.8, 10.425) -> (0.25, 10.425)
  line L726 (0.25, 10.425) -> (0.25, 10.875)
  line L727 (0.25, 10.875) -> (2.8, 10.875)
  line L728 (2.8, 12.075) -> (2.8, 11.625)
  line L729 (2.8, 11.625) -> (0.25, 11.625)
  line L730 (0.25, 11.625) -> (0.25, 12.075)
  line L731 (0.25, 12.075) -> (2.8, 12.075)
  line L732 (2.8, 13.275) -> (2.8, 12.825)
  line L733 (2.8, 12.825) -> (0.25, 12.825)
  line L734 (0.25, 12.825) -> (0.25, 13.275)
  line L735 (0.25, 13.275) -> (2.8, 13.275)
  line L736 (2.8, 14.475) -> (2.8, 14.025)
  line L737 (2.8, 14.025) -> (0.25, 14.025)
  line L738 (0.25, 14.025) -> (0.25, 14.475)
  line L739 (0.25, 14.475) -> (2.8, 14.475)
  line L740 (2.8, 15.675) -> (2.8, 15.225)
  line L741 (2.8, 15.225) -> (0.25, 15.225)
  line L742 (0.25, 15.225) -> (0.25, 15.675)
  line L743 (0.25, 15.675) -> (2.8, 15.675)
  line L744 (2.8, 21.075) -> (2.8, 20.625)
  line L745 (2.8, 20.625) -> (0.25, 20.625)
  line L746 (0.25, 20.625) -> (0.25, 21.075)
  line L747 (0.25, 21.075) -> (2.8, 21.075)
  line L748 (2.8, 22.275) -> (2.8, 21.825)
  line L749 (2.8, 21.825) -> (0.25, 21.825)
  line L750 (0.25, 21.825) -> (0.25, 22.275)
  line L751 (0.25, 22.275) -> (2.8, 22.275)
  line L752 (2.8, 23.475) -> (2.8, 23.025)
  line L753 (2.8, 23.025) -> (0.25, 23.025)
  line L754 (0.25, 23.025) -> (0.25, 23.475)
  line L755 (0.25, 23.475) -> (2.8, 23.475)
  line L756 (2.8, 24.675) -> (2.8, 24.225)
  line L757 (2.8, 24.225) -> (0.25, 24.225)
  line L758 (0.25, 24.225) -> (0.25, 24.675)
  line L759 (0.25, 24.675) -> (2.8, 24.675)
  line L760 (2.8, 25.875) -> (2.8, 25.425)
  line L761 (2.8, 25.425) -> (0.25, 25.425)
  line L762 (0.25, 25.425) -> (0.25, 25.875)
  line L763 (0.25, 25.875) -> (2.8, 25.875)
  line L764 (2.8, 27.075) -> (2.8, 26.625)
  line L765 (2.8, 26.625) -> (0.25, 26.625)
  line L766 (0.25, 26.625) -> (0.25, 27.075)
  line L767 (0.25, 27.075) -> (2.8, 27.075)
  line L768 (2.8, 28.275) -> (2.8, 27.825)
  line L769 (2.8, 27.825) -> (0.25, 27.825)
  line L770 (0.25, 27.825) -> (0.25, 28.275)
  line L771 (0.25, 28.275) -> (2.8, 28.275)
  line L772 (2.8, 29.475) -> (2.8, 29.025)
  line L773 (2.8, 29.025) -> (0.25, 29.025)
  line L774 (0.25, 29.025) -> (0.25, 29.475)
  line L775 (0.25, 29.475) -> (2.8, 29.475)
  line L776 (2.8, 30.675) -> (2.8, 30.225)
  line L777 (2.8, 30.225) -> (0.25, 30.225)
  line L778 (0.25, 30.225) -> (0.25, 30.675)
  line L779 (0.25, 30.675) -> (2.8, 30.675)
  line L780 (2.8, 16.275) -> (2.8, 15.825)
  line L781 (2.8, 15.825) -> (0.25, 15.825)
  line L782 (0.25, 15.825) -> (0.25, 16.275)
  line L783 (0.25, 16.275) -> (2.8, 16.275)
  line L784 (2.8, 31.875) -> (2.8, 31.425)
  line L785 (2.8, 31.425) -> (0.25, 31.425)
  line L786 (0.25, 31.425) -> (0.25, 31.875)
  line L787 (0.25, 31.875) -> (2.8, 31.875)
  line L788 (2.8, 31.275) -> (2.8, 30.825)
  line L789 (2.8, 30.825) -> (0.25, 30.825)
  line L790 (0.25, 30.825) -> (0.25, 31.275)
  line L791 (0.25, 31.275) -> (2.8, 31.275)
  line L792 (2.8, 30.075) -> (2.8, 29.625)
  line L793 (2.8, 29.625) -> (0.25, 29.625)
  line L794 (0.25, 29.625) -> (0.25, 30.075)
  line L795 (0.25, 30.075) -> (2.8, 30.075)
  line L796 (2.8, 28.875) -> (2.8, 28.425)
  line L797 (2.8, 28.425) -> (0.25, 28.425)
  line L798 (0.25, 28.425) -> (0.25, 28.875)
  line L799 (0.25, 28.875) -> (2.8, 28.875)
  line L800 (2.8, 27.675) -> (2.8, 27.225)
  line L801 (2.8, 27.225) -> (0.25, 27.225)
  line L802 (0.25, 27.225) -> (0.25, 27.675)
  line L803 (0.25, 27.675) -> (2.8, 27.675)
  line L804 (2.8, 26.475) -> (2.8, 26.025)
  line L805 (2.8, 26.025) -> (0.25, 26.025)
  line L806 (0.25, 26.025) -> (0.25, 26.475)
  line L807 (0.25, 26.475) -> (2.8, 26.475)
  line L808 (2.8, 25.275) -> (2.8, 24.825)
  line L809 (2.8, 24.825) -> (0.25, 24.825)
  line L810 (0.25, 24.825) -> (0.25, 25.275)
  line L811 (0.25, 25.275) -> (2.8, 25.275)
  line L812 (2.8, 24.075) -> (2.8, 23.625)
  line L813 (2.8, 23.625) -> (0.25, 23.625)
  line L814 (0.25, 23.625) -> (0.25, 24.075)
  line L815 (0.25, 24.075) -> (2.8, 24.075)
  line L816 (2.8, 22.875) -> (2.8, 22.425)
  line L817 (2.8, 22.425) -> (0.25, 22.425)
  line L818 (0.25, 22.425) -> (0.25, 22.875)
  line L819 (0.25, 22.875) -> (2.8, 22.875)
  line L820 (2.8, 21.675) -> (2.8, 21.225)
  line L821 (2.8, 21.225) -> (0.25, 21.225)
  line L822 (0.25, 21.225) -> (0.25, 21.675)
  line L823 (0.25, 21.675) -> (2.8, 21.675)
  line L824 (2.8, 20.475) -> (2.8, 20.025)
  line L825 (2.8, 20.025) -> (0.25, 20.025)
  line L826 (0.25, 20.025) -> (0.25, 20.475)
  line L827 (0.25, 20.475) -> (2.8, 20.475)
  line L828 (2.8, 15.075) -> (2.8, 14.625)
  line L829 (2.8, 14.625) -> (0.25, 14.625)
  line L830 (0.25, 14.625) -> (0.25, 15.075)
  line L831 (0.25, 15.075) -> (2.8, 15.075)
  line L832 (2.8, 13.875) -> (2.8, 13.425)
  line L833 (2.8, 13.425) -> (0.25, 13.425)
  line L834 (0.25, 13.425) -> (0.25, 13.875)
  line L835 (0.25, 13.875) -> (2.8, 13.875)
  line L836 (2.8, 12.675) -> (2.8, 12.225)
  line L837 (2.8, 12.225) -> (0.25, 12.225)
  line L838 (0.25, 12.225) -> (0.25, 12.675)
  line L839 (0.25, 12.675) -> (2.8, 12.675)
  line L840 (2.8, 11.475) -> (2.8, 11.025)
  line L841 (2.8, 11.025) -> (0.25, 11.025)
  line L842 (0.25, 11.025) -> (0.25, 11.475)
  line L843 (0.25, 11.475) -> (2.8, 11.475)
  line L844 (2.8, 10.275) -> (2.8, 9.825)
  line L845 (2.8, 9.825) -> (0.25, 9.825)
  line L846 (0.25, 9.825) -> (0.25, 10.275)
  line L847 (0.25, 10.275) -> (2.8, 10.275)
  line L848 (2.8, 9.075) -> (2.8, 8.625)
  line L849 (2.8, 8.625) -> (0.25, 8.625)
  line L850 (0.25, 8.625) -> (0.25, 9.075)
  line L851 (0.25, 9.075) -> (2.8, 9.075)
  line L852 (2.8, 7.875) -> (2.8, 7.425)
  line L853 (2.8, 7.425) -> (0.25, 7.425)
  line L854 (0.25, 7.425) -> (0.25, 7.875)
  line L855 (0.25, 7.875) -> (2.8, 7.875)
  line L856 (2.8, 6.675) -> (2.8, 6.225)
  line L857 (2.8, 6.225) -> (0.25, 6.225)
  line L858 (0.25, 6.225) -> (0.25, 6.675)
  line L859 (0.25, 6.675) -> (2.8, 6.675)
  line L860 (2.8, 5.475) -> (2.8, 5.025)
  line L861 (2.8, 5.025) -> (0.25, 5.025)
  line L862 (0.25, 5.025) -> (0.25, 5.475)
  line L863 (0.25, 5.475) -> (2.8, 5.475)
  line L864 (2.8, 4.275) -> (2.8, 3.825)
  line L865 (2.8, 3.825) -> (0.25, 3.825)
  line L866 (0.25, 3.825) -> (0.25, 4.275)
  line L867 (0.25, 4.275) -> (2.8, 4.275)
  line L868 (2.8, 3.075) -> (2.8, 2.625)
  line L869 (2.8, 2.625) -> (0.25, 2.625)
  line L870 (0.25, 2.625) -> (0.25, 3.075)
  line L871 (0.25, 3.075) -> (2.8, 3.075)
  line L872 (2.8, 1.875) -> (2.8, 1.425)
  line L873 (2.8, 1.425) -> (0.25, 1.425)
  line L874 (0.25, 1.425) -> (0.25, 1.875)
  line L875 (0.25, 1.875) -> (2.8, 1.875)
  line L876 (2.8, 0.675) -> (2.8, 0.225)
  line L877 (2.8, 0.225) -> (0.25, 0.225)
  line L878 (0.25, 0.225) -> (0.25, 0.675)
  line L879 (0.25, 0.675) -> (2.8, 0.675)
  line L880 (2.8, -0.525) -> (2.8, -0.975)
  line L881 (2.8, -0.975) -> (0.25, -0.975)
  line L882 (0.25, -0.975) -> (0.25, -0.525)
  line L883 (0.25, -0.525) -> (2.8, -0.525)
  line L884 (2.8, -1.725) -> (2.8, -2.175)
  line L885 (2.8, -2.175) -> (0.25, -2.175)
  line L886 (0.25, -2.175) -> (0.25, -1.725)
  line L887 (0.25, -1.725) -> (2.8, -1.725)
  line L888 (2.8, -2.925) -> (2.8, -3.375)
  line L889 (2.8, -3.375) -> (0.25, -3.375)
  line L890 (0.25, -3.375) -> (0.25, -2.925)
  line L891 (0.25, -2.925) -> (2.8, -2.925)
  line L892 (2.8, -4.125) -> (2.8, -4.575)
  line L893 (2.8, -4.575) -> (0.25, -4.575)
  line L894 (0.25, -4.575) -> (0.25, -4.125)
  line L895 (0.25, -4.125) -> (2.8, -4.125)
  line L896 (2.8, -5.325) -> (2.8, -5.775)
  line L897 (2.8, -5.775) -> (0.25, -5.775)
  line L898 (0.25, -5.775) -> (0.25, -5.325)
  line L899 (0.25, -5.325) -> (2.8, -5.325)
  line L900 (2.8, -6.525) -> (2.8, -6.975)
  line L901 (2.8, -6.975) -> (0.25, -6.975)
  line L902 (0.25, -6.975) -> (0.25, -6.525)
  line L903 (0.25, -6.525) -> (2.8, -6.525)
  line L904 (2.8, -7.725) -> (2.8, -8.175)
  line L905 (2.8, -8.175) -> (0.25, -8.175)
  line L906 (0.25, -8.175) -> (0.25, -7.725)
  line L907 (0.25, -7.725) -> (2.8, -7.725)
  line L908 (2.8, -8.925) -> (2.8, -9.375)
  line L909 (2.8, -9.375) -> (0.25, -9.375)
  line L910 (0.25, -9.375) -> (0.25, -8.925)
  line L911 (0.25, -8.925) -> (2.8, -8.925)
  line L912 (2.8, -10.125) -> (2.8, -10.575)
  line L913 (2.8, -10.575) -> (0.25, -10.575)
  line L914 (0.25, -10.575) -> (0.25, -10.125)
  line L915 (0.25, -10.125) -> (2.8, -10.125)
  line L916 (2.8, -11.325) -> (2.8, -11.775)
  line L917 (2.8, -11.775) -> (0.25, -11.775)
  line L918 (0.25, -11.775) -> (0.25, -11.325)
  line L919 (0.25, -11.325) -> (2.8, -11.325)
  line L920 (2.8, -12.525) -> (2.8, -12.975)
  line L921 (2.8, -12.975) -> (0.25, -12.975)
  line L922 (0.25, -12.975) -> (0.25, -12.525)
  line L923 (0.25, -12.525) -> (2.8, -12.525)
  line L924 (2.8, -13.725) -> (2.8, -14.175)
  line L925 (2.8, -14.175) -> (0.25, -14.175)
  line L926 (0.25, -14.175) -> (0.25, -13.725)
  line L927 (0.25, -13.725) -> (2.8, -13.725)
  line L928 (2.8, -14.925) -> (2.8, -15.375)
  line L929 (2.8, -15.375) -> (0.25, -15.375)
  line L930 (0.25, -15.375) -> (0.25, -14.925)
  line L931 (0.25, -14.925) -> (2.8, -14.925)
  line L932 (2.8, -16.125) -> (2.8, -16.575)
  line L933 (2.8, -16.575) -> (0.25, -16.575)
  line L934 (0.25, -16.575) -> (0.25, -16.125)
  line L935 (0.25, -16.125) -> (2.8, -16.125)
  line L936 (2.8, -17.325) -> (2.8, -17.775)
  line L937 (2.8, -17.775) -> (0.25, -17.775)
  line L938 (0.25, -17.775) -> (0.25, -17.325)
  line L939 (0.25, -17.325) -> (2.8, -17.325)
  line L940 (2.8, -18.525) -> (2.8, -18.975)
  line L941 (2.8, -18.975) -> (0.25, -18.975)
  line L942 (0.25, -18.975) -> (0.25, -18.525)
  line L943 (0.25, -18.525) -> (2.8, -18.525)
  line L944 (2.8, -19.725) -> (2.8, -20.175)
  line L945 (2.8, -20.175) -> (0.25, -20.175)
  line L946 (0.25, -20.175) -> (0.25, -19.725)
  line L947 (0.25, -19.725) -> (2.8, -19.725)
  line L948 (2.8, -20.925) -> (2.8, -21.375)
  line L949 (2.8, -21.375) -> (0.25, -21.375)
  line L950 (0.25, -21.375) -> (0.25, -20.925)
  line L951 (0.25, -20.925) -> (2.8, -20.925)
  line L952 (2.8, -22.125) -> (2.8, -22.575)
  line L953 (2.8, -22.575) -> (0.25, -22.575)
  line L954 (0.25, -22.575) -> (0.25, -22.125)
  line L955 (0.25, -22.125) -> (2.8, -22.125)
  line L956 (2.8, -23.325) -> (2.8, -23.775)
  line L957 (2.8, -23.775) -> (0.25, -23.775)
  line L958 (0.25, -23.775) -> (0.25, -23.325)
  line L959 (0.25, -23.325) -> (2.8, -23.325)
  line L960 (2.8, -24.525) -> (2.8, -24.975)
  line L961 (2.8, -24.975) -> (0.25, -24.975)
  line L962 (0.25, -24.975) -> (0.25, -24.525)
  line L963 (0.25, -24.525) -> (2.8, -24.525)
  line L964 (2.8, -25.725) -> (2.8, -26.175)
  line L965 (2.8, -26.175) -> (0.25, -26.175)
  line L966 (0.25, -26.175) -> (0.25, -25.725)
  line L967 (0.25, -25.725) -> (2.8, -25.725)
  line L968 (2.8, -26.925) -> (2.8, -27.375)
  line L969 (2.8, -27.375) -> (0.25, -27.375)
  line L970 (0.25, -27.375) -> (0.25, -26.925)
  line L971 (0.25, -26.925) -> (2.8, -26.925)
  line L972 (2.8, -28.125) -> (2.8, -28.575)
  line L973 (2.8, -28.575) -> (0.25, -28.575)
  line L974 (0.25, -28.575) -> (0.25, -28.125)
  line L975 (0.25, -28.125) -> (2.8, -28.125)
  line L976 (2.8, -29.325) -> (2.8, -29.775)
  line L977 (2.8, -29.775) -> (0.25, -29.775)
  line L978 (0.25, -29.775) -> (0.25, -29.325)
  line L979 (0.25, -29.325) -> (2.8, -29.325)
  line L980 (2.8, -30.525) -> (2.8, -30.975)
  line L981 (2.8, -30.975) -> (0.25, -30.975)
  line L982 (0.25, -30.975) -> (0.25, -30.525)
  line L983 (0.25, -30.525) -> (2.8, -30.525)
  arc A2 (0, -32.8) -> (1, -33.8) centre (1, -32.8) ccw
  line L984 (1, -33.8) -> (11.5, -33.8)
  arc A3 (12.5, -34.8) -> (11.5, -33.8) centre (11.5, -34.8) ccw
  line L985 (12.5, -34.8) -> (12.5, -45.4)
  line L986 (12.5, -45.4) -> (91.4, -45.4)
  line L987 (91.4, -45.4) -> (91.4, 45.4)
  line L988 (91.4, 45.4) -> (12.5, 45.4)
  line L989 (12.5, 45.4) -> (12.5, 34.8)
  arc A4 (11.5, 33.8) -> (12.5, 34.8) centre (11.5, 34.8) ccw
  line L990 (11.5, 33.8) -> (1, 33.8)
  arc A5 (1, 33.8) -> (0, 32.8) centre (1, 32.8) ccw
  line L991 (0, 32.8) -> (0, 18.95)
  line L992 (0, 18.95) -> (3.5, 18.95)
  arc A6 (3.5, 17.95) -> (3.5, 18.95) centre (3.5, 18.45) ccw
  line L993 (3.5, 17.95) -> (0, 17.95)
  line L994 (0, 17.95) -> (0, -32.8)
  line L995 (83.4, 15.4) -> (78.4, 15.4)
  line L996 (78.4, 15.4) -> (78.4, 14.6)
  line L997 (78.4, 14.6) -> (83.4, 14.6)
  line L998 (83.4, 14.6) -> (83.4, 15.4)
  line L999 (83.4, 14.6) -> (83.9, 14.6)
  line L1000 (83.4, -24.6) -> (78.4, -24.6)
  line L1001 (78.4, -24.6) -> (78.4, -25.4)
  line L1002 (78.4, -25.4) -> (83.4, -25.4)
  line L1003 (83.4, -25.4) -> (83.4, -24.6)
  line L1004 (83.4, -25.4) -> (83.9, -25.4)
  line L1005 (82.4, -23.9) -> (83.9, -23.9)
  line L1006 (83.9, -23.25) -> (83.9, -24.6)
  line L1007 (82.4, -26.1) -> (83.9, -26.1)
  line L1008 (83.9, -26.75) -> (83.9, -25.4)
  line L1009 (81.4, -20.1) -> (81.4, -23.9)
  line L1010 (81.4, -23.9) -> (77.9, -23.9)
  line L1011 (77.9, -23.9) -> (77.9, -26.1)
  line L1012 (82.4, -26.1) -> (81.4, -26.1)
  line L1013 (77.9, -26.1) -> (81.4, -26.1)
  line L1014 (82.4, 16.1) -> (83.9, 16.1)
  line L1015 (83.9, 16.75) -> (83.9, 15.4)
  line L1016 (82.4, 13.9) -> (83.9, 13.9)
  line L1017 (83.9, 14.6) -> (83.9, 13.25)
  line L1018 (81.4, 13.9) -> (81.4, 10.1)
  line L1019 (81.4, 13.9) -> (77.9, 13.9)
  line L1020 (77.9, 13.9) -> (77.9, 16.1)
  line L1021 (77.9, 16.1) -> (81.4, 16.1)
  line L1022 (12.8, 34.8) -> (12.8, 45.1)
  line L1023 (12.8, 45.1) -> (91.1, 45.1)
  line L1024 (91.1, 45.1) -> (91.1, -45.1)
  line L1025 (91.1, -45.1) -> (12.8, -45.1)
  line L1026 (12.8, -45.1) -> (12.8, -34.8)
  arc A7 (12.8, -34.8) -> (11.5, -33.5) centre (11.5, -34.8) ccw
  line L1027 (11.5, -33.5) -> (1, -33.5)
  arc A8 (0.3, -32.8) -> (1, -33.5) centre (1, -32.8) ccw
  line L1028 (0.3, -32.8) -> (0.3, 17.65)
  line L1029 (0.3, 17.65) -> (3.5, 17.65)
  arc A9 (3.5, 17.65) -> (3.5, 19.25) centre (3.5, 18.45) ccw
  line L1030 (3.5, 19.25) -> (0.3, 19.25)
  line L1031 (0.3, 19.25) -> (0.3, 32.8)
  arc A10 (1, 33.5) -> (0.3, 32.8) centre (1, 32.8) ccw
  line L1032 (1, 33.5) -> (11.5, 33.5)
  arc A11 (11.5, 33.5) -> (12.8, 34.8) centre (11.5, 34.8) ccw
  line L1033 (2.8, 23.625) -> (3.3, 23.625)
  arc A12 (3.3, 23.625) -> (3.575, 23.9) centre (3.3, 23.9) ccw
  line L1034 (3.575, 23.9) -> (3.575, 24.4)
  arc A13 (3.575, 24.4) -> (3.3, 24.675) centre (3.3, 24.4) ccw
  line L1035 (3.3, 24.675) -> (2.8, 24.675)
  line L1036 (2.8, 24.225) -> (2.8, 24.075)
  line L1037 (3.1, 33.5) -> (3.1, 24.975)
  line L1038 (3.1, 24.975) -> (3.3, 24.975)
  arc A14 (3.875, 24.4) -> (3.3, 24.975) centre (3.3, 24.4) ccw
  line L1039 (3.875, 24.4) -> (3.875, 23.9)
  arc A15 (3.3, 23.325) -> (3.875, 23.9) centre (3.3, 23.9) ccw
  line L1040 (3.3, 23.325) -> (3.1, 23.325)
  line L1041 (3.1, 23.325) -> (3.1, 19.25)
  circle A16 centre (3.3, 24.4) radius 0.175
  circle A17 centre (3.3, 23.9) radius 0.175
  line L1042 (2.8, -11.325) -> (2.8, -11.775) construction
  line L1043 (2.8, -11.55) -> (14.25, -11.55) construction
  line L1044 (14.25, -11.55) -> (17.25, -8.55) construction
  line L1045 (17.25, -8.55) -> (17.25, -6.35) construction
  line L1046 (2.8, -12.15) -> (14.3571, -12.15) construction
  line L1047 (14.3571, -12.15) -> (17.75, -8.7571) construction
  line L1048 (17.75, -8.7571) -> (17.75, -6.35) construction
  line L1049 (18.25, -6.35) -> (18.25, -8.9642) construction
  line L1050 (18.25, -8.9642) -> (14.4642, -12.75) construction
  line L1051 (14.4642, -12.75) -> (2.8, -12.75) construction
  line L1052 (2.8, -12.525) -> (2.8, -12.975) construction
  line L1053 (2.8, -13.35) -> (14.5713, -13.35) construction
  line L1054 (14.5713, -13.35) -> (18.75, -9.1713) construction
  line L1055 (18.75, -9.1713) -> (18.75, -6.35) construction
  line L1056 (3.1, 17.65) -> (3.1, -11.15)
  line L1057 (3.1, -33.5) -> (3.1, -13.75)
  line L1058 (17.15, -6.35) -> (17.15, -8.5086)
  line L1059 (17.15, -8.5086) -> (14.2086, -11.45)
  line L1060 (14.2086, -11.45) -> (2.8, -11.45)
  line L1061 (17.35, -6.35) -> (17.35, -8.5914)
  line L1062 (17.35, -8.5914) -> (14.2914, -11.65)
  line L1063 (14.2914, -11.65) -> (2.8, -11.65)
  line L1064 (17.65, -6.35) -> (17.65, -8.7157)
  line L1065 (17.65, -8.7157) -> (14.3157, -12.05)
  line L1066 (14.3157, -12.05) -> (2.8, -12.05)
  line L1067 (17.85, -6.35) -> (17.85, -8.7985)
  line L1068 (17.85, -8.7985) -> (14.3985, -12.25)
  line L1069 (14.3985, -12.25) -> (2.8, -12.25)
  line L1070 (18.15, -6.35) -> (18.15, -8.9228)
  line L1071 (18.15, -8.9228) -> (14.4228, -12.65)
  line L1072 (14.4228, -12.65) -> (2.8, -12.65)
  line L1073 (18.35, -6.35) -> (18.35, -9.0056)
  line L1074 (18.35, -9.0056) -> (14.5056, -12.85)
  line L1075 (14.5056, -12.85) -> (2.8, -12.85)
  line L1076 (18.65, -6.35) -> (18.65, -9.1299)
  line L1077 (18.65, -9.1299) -> (14.5299, -13.25)
  line L1078 (14.5299, -13.25) -> (2.8, -13.25)
  line L1079 (18.85, -6.35) -> (18.85, -9.2127)
  line L1080 (18.85, -9.2127) -> (14.6127, -13.45)
  line L1081 (14.6127, -13.45) -> (2.8, -13.45)
  line L1082 (17.1, -6.35) -> (17.4, -6.35)
  line L1083 (17.6, -6.35) -> (17.9, -6.35)
  line L1084 (18.1, -6.35) -> (18.4, -6.35)
  line L1085 (18.6, -6.35) -> (18.9, -6.35)
  line L1086 (2.8, -11.775) -> (2.8, -11.325)
  line L1087 (2.8, -12.375) -> (2.8, -11.925)
  line L1088 (2.8, -12.975) -> (2.8, -12.525)
  line L1089 (2.8, -13.575) -> (2.8, -13.125)
  line L1090 (23.75, -6.35) -> (23.75, -8.75) construction
  arc A18 (23.75, -8.75) -> (27.75, -12.75) centre (27.75, -8.75) ccw construction
  line L1091 (27.75, -12.75) -> (40.6, -12.75) construction
  line L1092 (23.25, -6.35) -> (23.25, -8.75) construction
  arc A19 (23.25, -8.75) -> (27.75, -13.25) centre (27.75, -8.75) ccw construction
  line L1093 (27.75, -13.25) -> (40.6, -13.25) construction
  line L1094 (40.6, -13) -> (27.75, -13) construction
  line L1095 (23.875, -6.35) -> (23.875, -8.75)
  arc A20 (23.875, -8.75) -> (27.75, -12.625) centre (27.75, -8.75) ccw
  line L1096 (27.75, -12.625) -> (40.6, -12.625)
  line L1097 (23.625, -6.35) -> (23.625, -8.75)
  arc A21 (23.625, -8.75) -> (27.75, -12.875) centre (27.75, -8.75) ccw
  line L1098 (27.75, -12.875) -> (40.6, -12.875)
  line L1099 (23.375, -6.35) -> (23.375, -8.75)
  arc A22 (23.375, -8.75) -> (27.75, -13.125) centre (27.75, -8.75) ccw
  line L1100 (27.75, -13.125) -> (40.6, -13.125)
  line L1101 (23.125, -6.35) -> (23.125, -8.75)
  arc A23 (23.125, -8.75) -> (27.75, -13.375) centre (27.75, -8.75) ccw
  line L1102 (27.75, -13.375) -> (40.6, -13.375)
  line L1103 (23.1, -6.35) -> (23.4, -6.35)
  line L1104 (23.6, -6.35) -> (23.9, -6.35)
  line L1105 (40.6, -12.625) -> (40.6, -12.875)
  line L1106 (40.6, -13.125) -> (40.6, -13.375)
  line L1107 (3.1, -13.75) -> (14.737, -13.75)
  line L1108 (14.737, -13.75) -> (19.15, -9.337)
  line L1109 (19.15, -9.337) -> (19.15, -6.65)
  line L1110 (19.15, -6.65) -> (22.4, -6.65)
  line L1111 (22.4, -6.65) -> (22.4, -8.75)